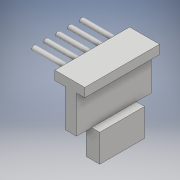
# Autodesk Inventor part: humidity_sensor_mount
Saved by Autodesk Inventor 2017.2 (Build 212233000, 233)
## iProperties
Created: 2017-10-12
Part Number: humidity_sensor_mount
Material: Generic
Document SubType Name: Modeling
Designer: Nic
Density: 1 g/cm^3
Appearance: Default
Author: Nic
Autodesk Inventor part; units mm, degrees
ref_plane "YZ Plane" through (0, 0, 0) normal (1, 0, 0) x (0, 1, 0)
ref_plane "XZ Plane" through (0, 0, 0) normal (0, 1, 0) x (-1, 0, 0)
ref_plane "XY Plane" through (0, 0, 0) normal (0, 0, 1) x (1, 0, 0)
sketch "Sketch1" plane through (0, 0, 0) normal (0, 1, 0) x (-1, 0, 0)
  line L0 (0, 0) -> (0, 3.7)
  line L1 (0, 3.7) -> (1.1, 3.7)
  line L2 (1.1, 8.7) -> (0, 8.7)
  line L3 (0, 8.7) -> (0, 9.9)
  line L4 (0, 9.9) -> (4, 9.9)
  line L5 (4, 9.9) -> (4, 8.7)
  line L6 (4, 8.7) -> (2.6, 8.7)
  line L7 (2.6, 8.7) -> (2.6, 3.7)
  line L8 (2.6, 3.7) -> (1.8, 3.7)
  line L9 (1.8, 3.7) -> (1.8, 0)
  line L10 (1.8, 0) -> (0, 0)
  line L11 (1.1, 3.7) -> (1.1, 8.7)
  dimension "d0" = 3.7
  dimension "d1" = 1.8
  dimension "d2" = 1.1
  dimension "d3" = 1.2
  dimension "d4" = 1.5
  dimension "d5" = 5
  dimension "d6" = 4
  constraints: 24 end point, 5 perpendicular, 3 horizontal, 3 point on line, 2 parallel, 2 vertical
  measures "d0" distance of L0.start L0.end
  measures "d1" distance of L9.end L0.start
  measures "d2" distance between parallel lines of L0 L11
  measures "d3" distance of L2.end L3.end
  measures "d4" distance between parallel lines of L11 L7
  measures "d5" distance between parallel lines of L1 L2
  measures "d6" distance between parallel lines of L3 L5
extrude "Extrusion1" add sketch "Sketch1" along normal blind 10
sketch "Sketch2" plane through (0, 0, 3.7) normal (1, 0, 0) x (0, 0, -1)
  line L0 (0, 0) -> (0, 10) projected
  line L1 (0, 0) -> (4, 0)
  line L2 (4, 0) -> (4, 2)
  line L3 (4, 2) -> (0, 2)
  line L4 (0, 2) -> (0, 0)
  line L5 (0, 5) -> (3.7, 5) construction
  line L6 (0, 10) -> (4, 10)
  line L7 (4, 10) -> (4, 8)
  line L8 (4, 8) -> (0, 8)
  line L9 (0, 8) -> (0, 10)
  point P0 (3.7, 0)
  dimension "d9" = 6
  dimension "d10" = 4
  constraints: 18 end point, 3 symmetric about line, 2 horizontal, 2 parallel, 1 midpoint, 1 perpendicular
  measures "d9" distance between parallel lines of L8 L3
  measures "d10" distance of L0.start L1.end
extrude "Extrusion2" cut sketch "Sketch2" against normal up to next
sketch "Sketch3" plane through (0, 8, 0) normal (0, 0, -1) x (-1, 0, 0)
  circle A0 centre (0.9, -1.12) radius 0.3
  circle A1 centre (0.9, -2.38) radius 0.3
  circle A2 centre (0.9, -3.64) radius 0.3
  circle A3 centre (0.9, -4.9) radius 0.3
  line L0 (0, -6) -> (1.8, -6) projected
  line L1 (0, -6) -> (0, 0) projected
  line L2 (0.9, -4.9) -> (0.9, -1.12) construction
  point P0 (0, -8)
  dimension "d13" = 0.6
  dimension "d14" = 1.26
  dimension "d15" = 1.26
  dimension "d16" = 1.26
  dimension "d17" = 1.1
  dimension "d18" = 0.9
  constraints: 4 centre point, 3 equal radius, 2 end point, 2 point on line, 1 vertical
  measures "d13" diameter of A0
  measures "d14" distance of A1.centre L2.end
  measures "d15" distance of A2.centre A1.centre
  measures "d16" distance of L2.start A2.centre
  measures "d17" distance from line of L0 L2.start
  measures "d18" distance from line of L1 L2.start
extrude "Extrusion3" cut sketch "Sketch3" against normal blind 3
sketch "Sketch4" plane through (-4, 0, 8.7) normal (-1, 0, 0) x (0, 0, 1)
  circle A0 centre (0.6, 8.2) radius 0.3
  circle A1 centre (0.6, 6.6) radius 0.3
  circle A2 centre (0.6, 5) radius 0.3
  circle A3 centre (0.6, 3.4) radius 0.3
  circle A4 centre (0.6, 1.8) radius 0.3
  line L0 (1.2, 0) -> (0, 0) projected
  line L1 (0.6, 0) -> (0.6, 9.9899) construction
  point P0 (-8.7, 0)
  dimension "d21" = 0.6
  dimension "d22" = 1.6
  dimension "d23" = 1.6
  dimension "d24" = 1.6
  dimension "d25" = 1.6
  dimension "d26" = 1.8
  constraints: 5 centre point, 5 point on line, 4 equal radius, 2 end point, 1 midpoint, 1 vertical
  measures "d21" diameter of A0
  measures "d22" distance of A1.centre A0.centre
  measures "d23" distance of A2.centre A1.centre
  measures "d24" distance of A3.centre A2.centre
  measures "d25" distance of A4.centre A3.centre
  measures "d26" distance from line of L0 A4.centre
extrude "Extrusion4" add sketch "Sketch4" along normal blind 4.6
body "Solid1"
